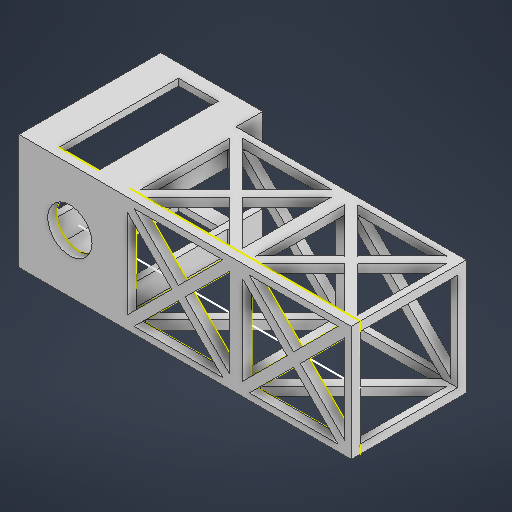
# Autodesk Inventor part: Part4
Saved by Autodesk Inventor 2026 (Build 300175000, 175)
## iProperties
Created: 2025-10-25
Part Number: Part4
Material: 一般
Document SubType Name: Modeling
Designer: masak
Density: 1 g/cm^3
Appearance: 既定
Author: masak
Autodesk Inventor part; units mm, degrees
ref_plane "YZ Plane" through (0, 0, 0) normal (1, 0, 0) x (0, 1, 0)
ref_plane "XZ Plane" through (0, 0, 0) normal (0, 1, 0) x (-1, 0, 0)
ref_plane "XY Plane" through (0, 0, 0) normal (0, 0, 1) x (1, 0, 0)
sketch "スケッチ1" plane through (0, 0, 0) normal (0, 0, 1) x (1, 0, 0)
  line L0 (0, -5) -> (-19, -5) projected
  line L1 (-19, 0) -> (-19, 12) projected
  line L2 (-19, 0) -> (-19, -5) projected
  line L3 (-19, 17) -> (-19, 12) projected
  line L4 (0, 17) -> (-19, 17) projected
  line L5 (0, 17) -> (0, 12) projected
  line L6 (0, 0) -> (0, 12) projected
  line L7 (0, 0) -> (0, -5) projected
  line L8 (-21, -7) -> (2, -7)
  line L9 (2, -7) -> (2, 19)
  line L10 (2, 19) -> (-21, 19)
  line L11 (-21, 19) -> (-21, -7)
  line L12 (-19, 4.1125) -> (-27, 4.1125) projected
  line L13 (-19, 7.8875) -> (-27, 7.8875) projected
  line L14 (0, 7.8875) -> (8, 7.8875) projected
  line L15 (0, 4.1125) -> (8, 4.1125) projected
  line L16 (-21, 19) -> (-21, 12)
  line L17 (-21, -7) -> (-21, 0)
  line L18 (2, 12) -> (0, 12)
  line L19 (2, 0) -> (0, 0)
  line L20 (2, -7) -> (-5, -7)
  line L21 (-21, -7) -> (-14, -7)
  line L22 (-5, 17) -> (-5, 19)
  line L23 (-14, 17) -> (-14, 19)
  line L24 (-21, 12) -> (-19, 12)
  line L25 (-21, 0) -> (-19, 0)
  line L26 (0, -7) -> (2, -5)
  line L27 (0, -5) -> (2, -7)
  line L28 (-20, 18) -> (1, 18)
  line L29 (1, 18) -> (1, -6)
  line L30 (1, -6) -> (-20, -6)
  line L31 (-20, -6) -> (-20, 18)
  line L32 (-20, 18) -> (-19, 17)
  line L33 (0, -5) -> (1, -6)
  line L34 (-19.5, 17.5) -> (0.5, 17.5)
  line L35 (0.5, 17.5) -> (0.5, -5.5)
  line L36 (0.5, -5.5) -> (-19.5, -5.5)
  line L37 (-19.5, -5.5) -> (-19.5, 17.5)
  line L38 (-14, -7) -> (-14, -5)
  line L39 (-5, -7) -> (-5, -5)
  point P0 (-21, 4.1125)
  point P1 (2, 4.1125)
  point P2 (2, 7.8875)
  point P3 (-21, 7.8875)
  point P4 (0.5, 12)
  point P5 (-19.5, 12)
  point P6 (0.5, 0)
  point P7 (-19.5, 0)
  point P8 (-14, -5.5)
  point P9 (-5, -5.5)
  point P10 (-14, 17.5)
  point P11 (-5, 17.5)
  dimension "d0" = 2
  dimension "d1" = 2
  dimension "d2" = 2
  dimension "d3" = 2
  dimension "d12" = 7
  dimension "d13" = 7
  dimension "d14" = 7
  dimension "d15" = 7
  constraints: 56 end point, 14 point on line, 10 perpendicular, 6 parallel, 4 horizontal, 3 midpoint
  measures "d0" distance between parallel lines of L11 L2
  measures "d1" distance from line of L10 L3.start
  measures "d2" distance from line of L9 L4.start
  measures "d3" distance from line of L8 L0.start
  measures "d12" distance of L10.end L16.end
  measures "d13" distance of L17.end L8.start
  measures "d14" distance of L21.end L8.start
  measures "d15" distance of L20.end L8.end
extrude "押し出し1" add sketch "スケッチ1" against normal blind 30 contours L35 L19 L29 L27 | L27 L30 L39 L36 | L27 L8 L26 | L29 L19 L9 L26 | L26 L9 L27 | L26 L8 L39 L30 | L38 L30 L31 L25 L37 L36 | L38 L8 L11 L25 L31 L30 | L35 L34 L22 L28 L29 L18 | L29 L28 L22 L10 L9 L18 | L24 L31 L32 L37 | L34 L32 L28 L23 | L24 L11 L10 L23 L28 L31
sketch "スケッチ2" plane through (0, 0, 0) normal (0, 0, 1) x (1, 0, 0)
  line L0 (-21, 19) -> (-21, -7) projected
  line L1 (2, 19) -> (2, -7) projected
  line L2 (-21, -7) -> (2, -7)
  line L3 (2, -7) -> (2, 19)
  line L4 (2, 19) -> (-21, 19)
  line L5 (-21, 19) -> (-21, -7)
  circle A0 centre (-9.5, 6) radius 5
  point P0 (0, 0)
  point P1 (-21, 4.1125)
  point P2 (2, 7.8875)
  point P3 (2, 7.8875)
  point P4 (-21, 4.1125)
  dimension "d11" = 10
  constraints: 8 end point, 2 parallel, 1 centre point, 1 horizontal, 1 perpendicular
  measures "d11" diameter of A0
extrude "押し出し2" add sketch "スケッチ2" along normal blind 2
sketch "スケッチ7" plane through (-14, -7, -30) normal (1, 0, 0) x (0, 0, -1)
  line L0 (0, 0) -> (-32, 0) projected
  line L1 (0, 7) -> (0, 0) projected
  line L2 (-30, 7) -> (0, 7) projected
  line L3 (-30, 7) -> (-30, 19) projected
  line L4 (-30, 19) -> (0, 19) projected
  line L5 (0, 26) -> (0, 19) projected
  line L6 (0, 26) -> (-32, 26) projected
  line L7 (-32, 0) -> (-32, 26) projected
  line L8 (0, 0) -> (-3, 0)
  line L9 (-3, 0) -> (-3, 26)
  line L10 (-3, 26) -> (0, 26)
  line L11 (0, 0) -> (0, 26)
  line L12 (-30, 19) -> (0, 19) projected
  line L13 (-3, 19) -> (0, 19)
  line L14 (-3, 7) -> (0, 7)
  line L15 (-30, 1.5) -> (0, 1.5) projected
  line L16 (-30, 24.5) -> (0, 24.5) projected
  point P0 (-30, 7)
  point P1 (-3, 1.5)
  point P2 (-3, 24.5)
  dimension "d21" = 3
  constraints: 12 end point, 6 point on line, 3 collinear, 2 perpendicular, 1 coincident
  measures "d21" distance of L11.start L8.end
extrude "押し出し6" add sketch "スケッチ7" along normal blind 10 contours L0 L9 L15 L1 | L6 L5 L16 L9
sketch "スケッチ8" plane through (2, -7, -30) normal (1, 0, 0) x (0, 0, -1)
  line L0 (0, 26) -> (-32, 26) projected
  line L1 (-32, 26) -> (-30, 26)
  line L2 (-30, 26) -> (-30, 0)
  line L3 (-30, 0) -> (-32, 0)
  line L4 (-32, 0) -> (-32, 26)
  point P0 (-30, 7)
  constraints: 8 end point, 2 parallel, 1 horizontal, 1 perpendicular
extrude "押し出し7" add sketch "スケッチ8" along normal blind 52
sketch "スケッチ9" plane through (0, 0, 0) normal (0, 0, -1) x (-1, 0, 0)
  line L0 (21, 19) -> (-2, 19) projected
  line L1 (-54, 19) -> (-54, -7) projected
  line L2 (-2, 19) -> (-54, 19)
  line L3 (-54, 19) -> (-54, -7)
  line L4 (-54, -7) -> (-2, -7)
  line L5 (-2, -7) -> (-2, 19)
  line L6 (-28, 19) -> (-28, -7)
  line L7 (-0.5, 17.5) -> (-0.5, 12) projected
  line L8 (-0.5, 17.5) -> (-54, 17.5)
  line L9 (-2, 19) -> (-28, -7)
  line L10 (-2, -7) -> (-28, 19)
  line L11 (-28, 19) -> (-54, -7)
  line L12 (-28, -7) -> (-54, 19)
  line L13 (-0.5, -5.5) -> (-0.5, 0) projected
  line L14 (-0.5, -5.5) -> (-54, -5.5)
  line L15 (-52.5, 17.5) -> (-52.5, -5.5)
  line L16 (-3.5, 17.5) -> (-3.5, -5.5)
  line L17 (-28, 17.5) -> (-52.5, -7)
  line L18 (-54, -5.5) -> (-29.5, 19)
  line L19 (-28, 17.5) -> (-3.5, -7)
  line L20 (-2, -5.5) -> (-26.5, 19)
  line L21 (-2, 17.5) -> (-26.5, -7)
  line L22 (-3.5, 19) -> (-28, -5.5)
  line L23 (-28, -5.5) -> (-51, 17.5)
  line L24 (-52.5, 16) -> (-29.5, -7)
  line L25 (-27.25, 17.5) -> (-28.9392, 17.5)
  line L26 (-28, 6.75) -> (-26.5, 6.75)
  line L27 (-26.5, 6.75) -> (-26.5, 19)
  line L28 (-26.5, 6.75) -> (-26.5, -7)
  line L29 (-29.5, 19) -> (-29.5, -7)
  point P0 (0, 0)
  point P1 (-41, 7.5)
  point P2 (-31, 17.5)
  point P3 (-42.5, 6)
  point P4 (-52.5, -4)
  point P5 (-31, -5.5)
  point P6 (-41, 4.5)
  point P7 (-51, -5.5)
  point P8 (-15, 7.5)
  point P9 (-5, 17.5)
  point P10 (-25, 17.5)
  point P11 (-16.5, 6)
  point P12 (-39.5, 6)
  point P13 (-15, 4.5)
  point P14 (-25, -5.5)
  point P15 (-5, -5.5)
  point P16 (-3.5, 16)
  point P17 (-13.5, 6)
  point P18 (-3.5, -4)
  point P19 (-26.5, -4)
  point P20 (-26.5, 16)
  point P21 (-29.5, -4)
  point P22 (-29.5, 16)
  constraints: 50 end point, 27 point on line, 10 perpendicular, 4 parallel, 2 midpoint, 1 collinear, 1 horizontal, 1 vertical, 10 other
extrude "押し出し8" cut sketch "スケッチ9" against normal blind 2 contours L18 L23 L8 | L24 L18 L15 | L29 L23 L17 | L17 L24 L14 | L8 L22 L20 | L19 L22 L28 L27 | L16 L20 L21 | L21 L19 L14
sketch "スケッチ10" plane through (0, 0, 0) normal (0, 0, -1) x (-1, 0, 0)
  line L0 (-3.5, 16) -> (-3.5, -4) projected
  line L1 (-3.5, -4) -> (-13.5, 6) projected
  line L2 (-13.5, 6) -> (-3.5, 16) projected
  line L3 (-42.5, 6) -> (-52.5, -4) projected
  line L4 (-52.5, -4) -> (-52.5, 16) projected
  line L5 (-52.5, 16) -> (-42.5, 6) projected
  line L6 (-31, -5.5) -> (-51, -5.5) projected
  line L7 (-51, -5.5) -> (-41, 4.5) projected
  line L8 (-41, 4.5) -> (-31, -5.5) projected
  line L9 (-26.5, 16) -> (-16.5, 6) projected
  line L10 (-16.5, 6) -> (-26.5, -4) projected
  line L11 (-26.5, -4) -> (-26.5, 16) projected
  line L12 (-15, 4.5) -> (-5, -5.5) projected
  line L13 (-5, -5.5) -> (-25, -5.5) projected
  line L14 (-25, -5.5) -> (-15, 4.5) projected
  line L15 (-51, 17.5) -> (-31, 17.5) projected
  line L16 (-31, 17.5) -> (-41, 7.5) projected
  line L17 (-41, 7.5) -> (-51, 17.5) projected
  line L18 (-15, 7.5) -> (-25, 17.5) projected
  line L19 (-25, 17.5) -> (-5, 17.5) projected
  line L20 (-5, 17.5) -> (-15, 7.5) projected
  line L21 (-29.5, -4) -> (-39.5, 6) projected
  line L22 (-39.5, 6) -> (-29.5, 16) projected
  line L23 (-29.5, 16) -> (-29.5, -4) projected
  line L24 (5, -5.5) -> (5, -7) projected
  line L25 (14, -7) -> (5, -7) projected
  line L26 (14, -7) -> (14, -5.5) projected
  line L27 (14, -5.5) -> (19.5, -5.5) projected
  line L28 (19.5, -5.5) -> (19.5, 0) projected
  line L29 (19.5, 0) -> (21, 0) projected
  line L30 (21, 12) -> (21, 0) projected
  line L31 (21, 12) -> (19.5, 12) projected
  line L32 (19.5, 12) -> (19.5, 17.5) projected
  line L33 (19.5, 17.5) -> (14, 17.5) projected
  line L34 (14, 17.5) -> (14, 19) projected
  line L35 (5, 19) -> (14, 19) projected
  line L36 (5, 19) -> (5, 17.5) projected
  line L37 (5, 17.5) -> (-0.5, 17.5) projected
  line L38 (-0.5, 17.5) -> (-0.5, 12) projected
  line L39 (-0.5, 12) -> (-2, 12) projected
  line L40 (-2, 19) -> (-2, 12) projected
  line L41 (-2, 19) -> (-54, 19) projected
  line L42 (-54, -7) -> (-54, 19) projected
  line L43 (-2, -7) -> (-54, -7) projected
  line L44 (-2, 0) -> (-2, -7) projected
  line L45 (-2, 0) -> (-0.5, 0) projected
  line L46 (-0.5, 0) -> (-0.5, -5.5) projected
  line L47 (-0.5, -5.5) -> (5, -5.5) projected
  circle A0 centre (9.5, 6) radius 5 projected
  line L48 (-2, 17.5) -> (-3.5, 17.5)
  line L49 (-3.5, 17.5) -> (-3.5, 19)
  line L50 (-26.5, 17.5) -> (-29.5, 17.5)
  line L51 (-29.5, 17.5) -> (-29.5, 19)
  line L52 (-26.5, 17.5) -> (-26.5, 19)
  line L53 (-52.5, 19) -> (-52.5, 17.5)
  line L54 (-52.5, 17.5) -> (-54, 17.5)
  line L55 (9.5, 6) -> (-54, 6)
  line L56 (-2, -7) -> (-2, 0)
  line L57 (-2, -7) -> (-54, -7)
  line L58 (-2, -5.5) -> (-3.5, -5.5)
  line L59 (-3.5, -5.5) -> (-3.5, -7)
  line L60 (-26.5, -5.5) -> (-29.5, -5.5)
  line L61 (-29.5, -5.5) -> (-29.5, -7)
  line L62 (-26.5, -5.5) -> (-26.5, -7)
  line L63 (-52.5, -7) -> (-52.5, -5.5)
  line L64 (-52.5, -5.5) -> (-54, -5.5)
  point P0 (0, 0)
  constraints: 34 end point, 19 point on line, 10 symmetric about line, 1 horizontal, 1 midpoint, 1 parallel, 1 perpendicular
sketch "スケッチ11" plane through (-21, 19, -30) normal (0, 1, 0) x (1, 0, 0)
  line L0 (24.5, -30) -> (24.5, -32) projected
  line L1 (23, -30) -> (75, -30) projected
  line L2 (36, -30) -> (36, -32) projected
  line L3 (23, -30) -> (36, -30)
  line L4 (0, -32) -> (75, -32) projected
  line L5 (23, -32) -> (23, -6)
  line L6 (23, -6) -> (75, -6)
  line L7 (75, -6) -> (75, -32)
  line L8 (23, -6) -> (23, -7.5)
  line L9 (23, -7.5) -> (75, -7.5)
  line L10 (73.5, -30) -> (73.5, -32) projected
  line L11 (73.5, -30) -> (73.5, -6)
  line L12 (24.5, -30) -> (24.5, -6)
  line L13 (49, -30) -> (49, -6)
  line L14 (49, -30) -> (49, -32)
  line L15 (23, -6) -> (49, -32)
  line L16 (75, -6) -> (49, -32)
  line L17 (49, -6) -> (23, -32)
  line L18 (49, -6) -> (75, -32)
  line L19 (24.5, -6) -> (49, -30.5)
  line L20 (73.5, -6) -> (49, -30.5)
  line L21 (50.5, -32) -> (75, -7.5)
  line L22 (47.5, -32) -> (23, -7.5)
  line L23 (24.5, -32) -> (49, -7.5)
  line L24 (49, -7.5) -> (73.5, -32)
  line L25 (75, -30.5) -> (50.5, -6)
  line L26 (47.5, -6) -> (23, -30.5)
  line L27 (47.5, -7.5) -> (47.5, -30.5)
  line L28 (50.5, -7.5) -> (50.5, -30.5)
  point P0 (21, -30)
  point P1 (73.5, -29)
  point P2 (63.5, -19)
  point P3 (73.5, -9)
  point P4 (52, -7.5)
  point P5 (72, -7.5)
  point P6 (62, -17.5)
  point P7 (46, -7.5)
  point P8 (36, -17.5)
  point P9 (26, -7.5)
  point P10 (26.5, -30)
  point P11 (36, -20.5)
  point P12 (45.5, -30)
  point P13 (48.5, -30)
  point P14 (37.5, -19)
  point P15 (60.5, -19)
  point P16 (49.5, -30)
  point P17 (52.5, -30)
  point P18 (62, -20.5)
  point P19 (71.5, -30)
  point P20 (34.5, -19)
  point P21 (24.5, -29)
  point P22 (24.5, -9)
  point P23 (50.5, -29)
  point P24 (50.5, -9)
  point P25 (47.5, -9)
  point P26 (47.5, -29)
  dimension "d28" = 26
  dimension "d29" = 1.5
  constraints: 48 end point, 22 point on line, 7 perpendicular, 3 parallel, 2 horizontal, 2 midpoint, 1 collinear, 1 vertical, 5 other
  measures "d28" distance of L5.start L5.end
  measures "d29" distance of L5.end L8.end
extrude "押し出し9" add sketch "スケッチ11" against normal blind 2 contours L12 L26 L22 L17 L1 | L1 L26 L12 | L1 L5 L22 L12 L26 | L17 L22 L23 L1 | L22 L26 L15 L17 | L17 L15 L23 L22 | L22 L9 L12 | L12 L15 L26 L22 | L5 L15 L9 | L23 L15 L1 L22 | L17 L19 L23 L15 | L15 L26 L19 L17 | L12 L19 L9 | L15 L6 L12 | L9 L19 L26 L15 | L23 L19 L27 L1 L15 | L19 L26 L9 L17 | L17 L27 L23 L19 | L19 L6 L26 L9 | L17 L13 L9 | L9 L26 L6 L17 | L9 L23 L27 | L27 L19 L1 | L27 L23 L13 L1 L19 | L13 L18 L9 | L24 L28 L20 L1 L13 | L9 L28 L24 | L6 L25 L9 L18 | L1 L16 L24 L21 | L20 L28 L1 | L1 L28 L20 L24 L16 | L9 L25 L20 L18 | L18 L20 L24 L28 | L6 L20 L9 L25 | L24 L21 L18 L1 | L24 L16 L18 L21 | L24 L20 L18 L16 | L20 L25 L16 L18 | L6 L16 L11 | L11 L9 L20 | L11 L25 L1 | L1 L18 L21 L25 L11 | L18 L16 L25 L21 | L9 L16 L25 L20 | L7 L9 L16 | L9 L21 L11 | L11 L21 L25 L16 | L1 L25 L11 L21 L7
sketch "スケッチ12" plane through (-21, -7, -30) normal (0, -1, 0) x (1, 0, 0)
  line L0 (24.5, 29) -> (34.5, 19) projected
  line L1 (34.5, 19) -> (24.5, 9) projected
  line L2 (24.5, 9) -> (24.5, 29) projected
  line L3 (36, 20.5) -> (26.5, 30) projected
  line L4 (45.5, 30) -> (36, 20.5) projected
  line L5 (37.5, 19) -> (47.5, 29) projected
  line L6 (47.5, 29) -> (47.5, 9) projected
  line L7 (47.5, 9) -> (37.5, 19) projected
  line L8 (36, 17.5) -> (46, 7.5) projected
  line L9 (46, 7.5) -> (26, 7.5) projected
  line L10 (23, 6) -> (75, 6) projected
  line L11 (26, 7.5) -> (36, 17.5) projected
  line L12 (50.5, 9) -> (50.5, 29) projected
  line L13 (60.5, 19) -> (50.5, 9) projected
  line L14 (52, 7.5) -> (62, 17.5) projected
  line L15 (72, 7.5) -> (52, 7.5) projected
  line L16 (62, 17.5) -> (72, 7.5) projected
  line L17 (73.5, 9) -> (63.5, 19) projected
  line L18 (73.5, 29) -> (73.5, 9) projected
  line L19 (63.5, 19) -> (73.5, 29) projected
  line L20 (71.5, 30) -> (62, 20.5) projected
  line L21 (62, 20.5) -> (52.5, 30) projected
  line L22 (50.5, 29) -> (60.5, 19) projected
  line L23 (75, 6) -> (75, 30) projected
  line L24 (45.5, 30) -> (52.5, 30) projected
  line L25 (45.5, 30) -> (36, 20.5) projected
  line L26 (36, 20.5) -> (26.5, 30) projected
  line L27 (23, 30) -> (26.5, 30) projected
  line L28 (23, 6) -> (23, 30) projected
  line L29 (23, 6) -> (75, 6) projected
  line L30 (75, 6) -> (75, 30) projected
  line L31 (71.5, 30) -> (75, 30) projected
  line L32 (71.5, 30) -> (62, 20.5) projected
  line L33 (62, 20.5) -> (52.5, 30) projected
  line L34 (63.5, 19) -> (73.5, 29) projected
  line L35 (73.5, 29) -> (73.5, 9) projected
  line L36 (73.5, 9) -> (63.5, 19) projected
  line L37 (72, 7.5) -> (52, 7.5) projected
  line L38 (52, 7.5) -> (62, 17.5) projected
  line L39 (62, 17.5) -> (72, 7.5) projected
  line L40 (36, 17.5) -> (46, 7.5) projected
  line L41 (46, 7.5) -> (26, 7.5) projected
  line L42 (26, 7.5) -> (36, 17.5) projected
  line L43 (24.5, 29) -> (34.5, 19) projected
  line L44 (34.5, 19) -> (24.5, 9) projected
  line L45 (24.5, 9) -> (24.5, 29) projected
  line L46 (47.5, 29) -> (47.5, 9) projected
  line L47 (47.5, 9) -> (37.5, 19) projected
  line L48 (37.5, 19) -> (47.5, 29) projected
  line L49 (60.5, 19) -> (50.5, 9) projected
  line L50 (50.5, 9) -> (50.5, 29) projected
  line L51 (50.5, 29) -> (60.5, 19) projected
  point P0 (21, 30)
extrude "押し出し10" add sketch "スケッチ12" against normal blind 2
sketch "スケッチ13" plane through (54, 19, -24) normal (0, 0, -1) x (-1, 0, 0)
  line L0 (48.5, -24) -> (52, -24) projected
  line L1 (52, -19) -> (52, -24) projected
  line L2 (52, -19) -> (53.5, -19) projected
  line L3 (53.5, -19) -> (53.5, -24.5) projected
  line L4 (53.5, -24.5) -> (59, -24.5) projected
  line L5 (59, -24.5) -> (59, -26) projected
  line L6 (68, -26) -> (59, -26) projected
  line L7 (68, -26) -> (68, -24.5) projected
  line L8 (68, -24.5) -> (73.5, -24.5) projected
  line L9 (73.5, -24.5) -> (73.5, -19) projected
  line L10 (73.5, -19) -> (75, -19) projected
  line L11 (75, -7) -> (75, -19) projected
  line L12 (75, -7) -> (73.5, -7) projected
  line L13 (73.5, -7) -> (73.5, -1.5) projected
  line L14 (73.5, -1.5) -> (68, -1.5) projected
  line L15 (68, -1.5) -> (68, 0) projected
  line L16 (59, 0) -> (68, 0) projected
  line L17 (59, 0) -> (59, -1.5) projected
  line L18 (59, -1.5) -> (53.5, -1.5) projected
  line L19 (53.5, -1.5) -> (53.5, -7) projected
  line L20 (53.5, -7) -> (52, -7) projected
  line L21 (52, -2) -> (52, -7) projected
  line L22 (52, -2) -> (48.5, -2) projected
  line L23 (48.5, -2) -> (39, -11.5) projected
  line L24 (39, -11.5) -> (29.5, -2) projected
  line L25 (29.5, -2) -> (22.5, -2) projected
  line L26 (22.5, -2) -> (13, -11.5) projected
  line L27 (13, -11.5) -> (3.5, -2) projected
  line L28 (3.5, -2) -> (0, -2) projected
  line L29 (0, -24) -> (0, -2) projected
  line L30 (0, -24) -> (3.5, -24) projected
  line L31 (3.5, -24) -> (13, -14.5) projected
  line L32 (13, -14.5) -> (22.5, -24) projected
  line L33 (22.5, -24) -> (29.5, -24) projected
  line L34 (29.5, -24) -> (39, -14.5) projected
  line L35 (39, -14.5) -> (48.5, -24) projected
  circle A0 centre (63.5, -13) radius 5 projected
  line L36 (24.5, -23) -> (14.5, -13) projected
  line L37 (14.5, -13) -> (24.5, -3) projected
  line L38 (24.5, -3) -> (24.5, -23) projected
  line L39 (27.5, -3) -> (37.5, -13) projected
  line L40 (37.5, -13) -> (27.5, -23) projected
  line L41 (27.5, -23) -> (27.5, -3) projected
  line L42 (11.5, -13) -> (1.5, -23) projected
  line L43 (1.5, -23) -> (1.5, -3) projected
  line L44 (1.5, -3) -> (11.5, -13) projected
  line L45 (50.5, -3) -> (50.5, -23) projected
  line L46 (50.5, -23) -> (40.5, -13) projected
  line L47 (40.5, -13) -> (50.5, -3) projected
  line L48 (52, -7) -> (52, -19)
  point P0 (54, -19)
  constraints: 2 end point, 1 parallel
extrude "押し出し11" add sketch "スケッチ13" against normal blind 2 contours L35 L34 L33 L32 L31 L30 L29 L28 L27 L26 L25 L24 L23 L22 L21 L48 L1 L0
sketch "スケッチ14" plane through (54, -7, -24) normal (0, 0, -1) x (-1, 0, 0)
  line L0 (52, 7) -> (52, 19) projected
  line L1 (53.5, 7) -> (52, 7) projected
  line L2 (52, 19) -> (52, 7)
  line L3 (52, 7) -> (50.5, 7)
  line L4 (50.5, 23) -> (50.5, 3) projected
  line L5 (52, 19) -> (50.5, 19)
  line L6 (50.5, 19) -> (50.5, 7)
  point P0 (54, 7)
  constraints: 8 end point, 2 perpendicular, 1 horizontal, 1 point on line, 1 vertical
extrude "押し出し12" cut sketch "スケッチ14" against normal blind 2
